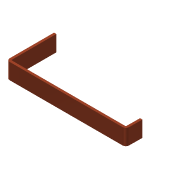
# Autodesk Inventor part: 17-0028-0119
Saved by Autodesk Inventor 2016 SP2 (Build 200236200, 236)
## iProperties
Category: IOP
Company: Universiteit van Amsterdam
Created: 2018-07-20
Part Number: 17-0028-0119
Material: Copper
Document SubType Name: Modeling
Designer: Daan Giesen
Density: 8.94 g/cm^3
Appearance: Copper - Satin
User Status: Work in Progress
Authority: Reichsöllner, Lukas
Cost Center: 17-0028
Author: Daan Giesen
Revision Number: A
Autodesk Inventor part; units mm, degrees
ref_plane "YZ Plane" through (0, 0, 0) normal (1, 0, 0) x (0, 1, 0)
ref_plane "XZ Plane" through (0, 0, 0) normal (0, 1, 0) x (-1, 0, 0)
ref_plane "XY Plane" through (0, 0, 0) normal (0, 0, 1) x (1, 0, 0)
sketch "Sketch1" plane through (0, 0, 0) normal (0, 0, 1) x (1, 0, 0)
  line L0 (0, 138) -> (0, -23) construction
  line L1 (-361.2743, 0) -> (60.6456, 0) construction
  line L2 (0, 0) -> (0.3713, 41.5996)
  line L3 (0.3713, 41.5996) -> (-5.6284, 41.6531)
  line L4 (-5.6284, 41.6531) -> (-5.9467, 6)
  line L5 (-5.9467, 6) -> (-295, 6)
  line L6 (-295, 6) -> (-295, 115)
  line L7 (-295, 115) -> (-301, 115)
  line L8 (-301, 115) -> (-301, 0)
  line L9 (0, 0) -> (-301, 0)
  dimension "d4" = 41.5996
  dimension "d5" = 301
  dimension "d6" = 115
  dimension "d7" = 6
  dimension "d8" = 6
  dimension "d9" = 6
  constraints: 16 end point, 5 perpendicular, 1 collinear, 1 point on line, 1 vertical
  measures "d4" vertical distance of L2.start L2.end
  measures "d5" distance of L2.start L8.end
  measures "d6" distance of L7.end L8.end
  measures "d7" distance between parallel lines of L8 L6
  measures "d8" distance between parallel lines of L9 L5
  measures "d9" distance between parallel lines of L2 L4
extrude "Extrusion3" add sketch "Sketch1" along normal blind 40
fillet "Fillet1" radius 2 2 edges at (-5.9467, 6, 20) (-295, 6, 20)
fillet "Fillet2" radius 8 2 edges at (0, 0, 20) (-301, 0, 20)
equation "\"d8\" = d7"
equation "\"d9\" = d7"
body "Solid3"
